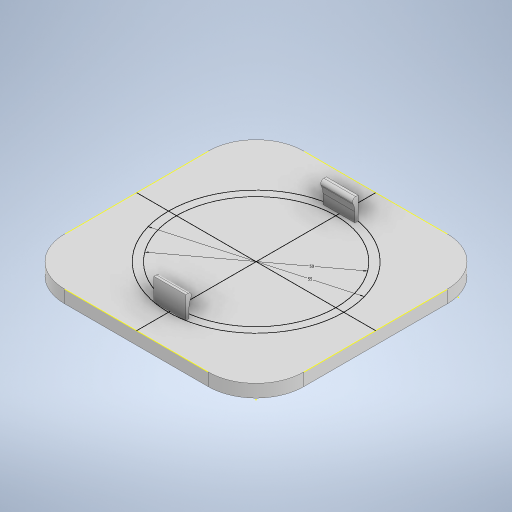
# Autodesk Inventor part: cone_p1_testpart1
Saved by Autodesk Inventor 2024 (Build 280153000, 153)
## iProperties
Created: 2023-09-27
Part Number: cone_p1_testpart1
Material: Generic
Document SubType Name: Modeling
Designer: kubad
Density: 1 g/cm^3
Appearance: Default
Author: kubad
## iProperties of the stored document cone_p1_testpart1_3DPrint.ipt
Created: 2023-09-28
Part Number: cone_p1_testpart1_3DPrint
Material: Generic
Document SubType Name: Modeling
Designer: kubad
Density: 1 g/cm^3
Appearance: Default
Author: kubad
Autodesk Inventor part; units mm, degrees
ref_plane "YZ Plane" through (0, 0, 0) normal (1, 0, 0) x (0, 1, 0)
ref_plane "XZ Plane" through (0, 0, 0) normal (0, 1, 0) x (-1, 0, 0)
ref_plane "XY Plane" through (0, 0, 0) normal (0, 0, 1) x (1, 0, 0)
sketch "Sketch1" plane through (0, 0, 0) normal (0, 1, 0) x (-1, 0, 0)
  line L0 (0, 0) -> (75, 0)
  line L1 (75, 0) -> (75, -75)
  line L2 (75, -75) -> (0, -75)
  line L3 (0, -75) -> (0, 0)
  dimension "d0" = 75
  dimension "d1" = 75
  constraints: 8 end point, 2 parallel, 1 horizontal, 1 perpendicular
  measures "d0" distance of L1.end L2.end
  measures "d1" distance of L0.end L1.end
extrude "Extrusion1" add sketch "Sketch1" along normal blind 4
sketch "Sketch2" plane through (0, 4, 0) normal (0, 1, 0) x (1, 0, 0)
  line L0 (-75, 75) -> (-75, 0) projected
  line L1 (-75, 37.5) -> (0, 37.5)
  line L2 (0, 75) -> (-75, 75) projected
  line L3 (-37.5, 75) -> (-37.5, 0)
  line L4 (-75, 0) -> (0, 0) projected
  circle A0 centre (-37.5, 37.5) radius 22.5
  circle A1 centre (-37.5, 37.5) radius 27.5
  line L5 (-37.5, 10) -> (-42.5, 10)
  line L6 (-42.5, 10.4584) -> (-32.5, 10.4584)
  line L7 (-32.5, 10.4584) -> (-32.5, 11.4584)
  line L8 (-32.5, 11.4584) -> (-42.5, 11.4584)
  line L9 (-42.5, 11.4584) -> (-42.5, 10.4584)
  line L10 (-37.5, 65) -> (-42.5, 65)
  line L11 (-42.5, 64.5416) -> (-32.5, 64.5416)
  line L12 (-32.5, 64.5416) -> (-32.5, 63.5416)
  line L13 (-32.5, 63.5416) -> (-42.5, 63.5416)
  line L14 (-42.5, 63.5416) -> (-42.5, 64.5416)
  line L15 (-42.5, 10.4584) -> (-32.5, 10.4584)
  line L16 (-32.5, 10.4584) -> (-32.5, 11.4584)
  line L17 (-32.5, 11.4584) -> (-42.5, 11.4584)
  line L18 (-42.5, 11.4584) -> (-42.5, 10.4584)
  dimension "d4" = 45
  dimension "d5" = 55
  dimension "d6" = 5
  dimension "d7" = 10
  dimension "d8" = 1
  dimension "d9" = 5
  dimension "d10" = 10
  dimension "d11" = 1
  constraints: 32 end point, 6 parallel, 5 horizontal, 4 midpoint, 4 perpendicular, 4 point on circle, 2 centre point, 1 coincident, 1 point on line, 1 tangent
  measures "d4" diameter of A0
  measures "d5" diameter of A1
  measures "d6" distance of L5.start L5.end
  measures "d7" distance of L8.end L7.end
  measures "d8" distance of L7.end L6.end
  measures "d9" distance of L10.start L10.end
  measures "d10" distance of L12.end L13.end
  measures "d11" distance of L11.end L12.end
extrude "Extrusion2" add sketch "Sketch2" along normal blind 7 contours L11 L3 L13 L14 | L9 L8 L3 L6 | L11 L12 L13 L3 | L3 L8 L7 L6
sketch "Sketch3" plane through (-42.5, 4, -63.5416) normal (0, 0, 1) x (1, 0, 0)
  point P0 (42.5, -4)
sketch "Sketch4" plane through (-42.5, 4, -63.5416) normal (0, 0, 1) x (1, 0, 0)
  line L0 (10, 7) -> (0, 7) projected
  line L1 (10, 0) -> (10, 7) projected
  line L2 (0, 7) -> (10, 7)
  line L3 (10, 7) -> (10, 6)
  line L4 (10, 6) -> (0, 6)
  line L5 (0, 6) -> (0, 7)
  point P0 (42.5, -4)
  dimension "d14" = 1
  constraints: 8 end point, 2 parallel, 1 horizontal, 1 perpendicular, 1 point on line
  measures "d14" distance of L2.end L3.end
extrude "Extrusion3" add sketch "Sketch4" along normal blind 1
sketch "Sketch5" plane through (-32.5, 4, -11.4584) normal (0, 0, -1) x (-1, 0, 0)
  line L0 (0, 7) -> (10, 7) projected
  line L1 (10, 0) -> (10, 7) projected
  line L2 (0, 7) -> (10, 7)
  line L3 (10, 7) -> (10, 6)
  line L4 (10, 6) -> (0, 6)
  line L5 (0, 6) -> (0, 7)
  point P0 (-32.5, -4)
  dimension "d17" = 1
  constraints: 8 end point, 2 parallel, 1 horizontal, 1 perpendicular, 1 point on line
  measures "d17" distance of L2.end L3.end
extrude "Extrusion4" add sketch "Sketch5" along normal blind 1
fillet "Fillet1" radius 5 1 edges at (-37.5, 10, -63.5416)
fillet "Fillet2" radius 5 1 edges at (-37.5, 10, -11.4584)
fillet "Fillet3" radius 5 2 edges at (-37.5, 10, -62.5416) (-37.5, 10, -12.4584)
fillet "Fillet4" radius 1 2 edges at (-37.5, 11, -62.5416) (-37.5, 11, -12.4584)
fillet "Fillet5" radius 15 4 edges at (0, 2, 0) (-75, 2, 0) (-75, 2, -75) (0, 2, -75)
sketch "Sketch6" plane through (0, 4, 0) normal (0, 1, 0) x (1, 0, 0)
  line L0 (0, 15) -> (0, 60) projected
  line L1 (0, 37.5) -> (-75, 37.5)
  line L2 (-75, 60) -> (-75, 15) projected
  line L3 (-60, 0) -> (-15, 0) projected
  line L4 (-37.5, 0) -> (-37.5, 75)
  line L5 (-15, 75) -> (-60, 75) projected
  circle A0 centre (-37.5, 37.5) radius 27.5
  circle A1 centre (-37.5, 37.5) radius 25
  point P0 (0, 0)
  dimension "d27" = 55
  dimension "d28" = 50
  constraints: 5 midpoint, 4 end point, 2 centre point, 1 coincident
  measures "d27" diameter of A0
  measures "d28" diameter of A1
sketch "Sketch7" plane through (0, 4, 0) normal (0, 1, 0) x (1, 0, 0)
  point P0 (0, 0)
sketch "Sketch8" plane through (0, 4, 0) normal (0, 1, 0) x (1, 0, 0)
  point P0 (0, 0)
body "Solid1"
